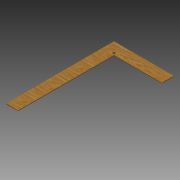
# Autodesk Inventor part: stand_plate1
Saved by Autodesk Inventor 2013 (Build 170138000, 138)
## iProperties
Created: 2014-10-20
Part Number: stand_plate1
Material: Plywood, Finish
Document SubType Name: Modeling
Designer: Masta
Density: 1 g/cm^3
Author: Masta
Autodesk Inventor part; units mm, degrees
ref_plane "YZ Plane" through (0, 0, 0) normal (1, 0, 0) x (0, 1, 0)
ref_plane "XZ Plane" through (0, 0, 0) normal (0, 1, 0) x (-1, 0, 0)
ref_plane "XY Plane" through (0, 0, 0) normal (0, 0, 1) x (1, 0, 0)
sketch "Sketch1" plane through (0, 0, 0) normal (0, 0, 1) x (1, 0, 0)
  line L0 (0, 0) -> (500, 0)
  line L1 (500, 0) -> (500, -100)
  line L2 (500, -100) -> (100, -100)
  line L3 (100, -100) -> (100, -900)
  line L4 (100, -900) -> (0, -900)
  line L5 (0, -900) -> (0, 0)
  line L6 (100, -100) -> (85, -100) construction
  line L7 (85, -100) -> (85, -85) construction
  dimension "d0" = 500
  dimension "d1" = 100
  dimension "d2" = 400
  dimension "d3" = 800
  dimension "d6" = 15
  constraints: 16 end point, 6 perpendicular, 2 parallel, 1 coincident, 1 horizontal
  measures "d0" distance of L0.start L0.end
  measures "d1" distance of L0.end L1.end
  measures "d2" distance of L1.end L2.end
  measures "d3" distance of L2.end L3.end
  measures "d6" distance of L2.end L6.end
extrude "Extrusion1" add sketch "Sketch1" along normal blind 5
hole "Hole1" at (85, -85, 0) direction (0, 0, 1) diameter 20 end through all
body "Solid1"
